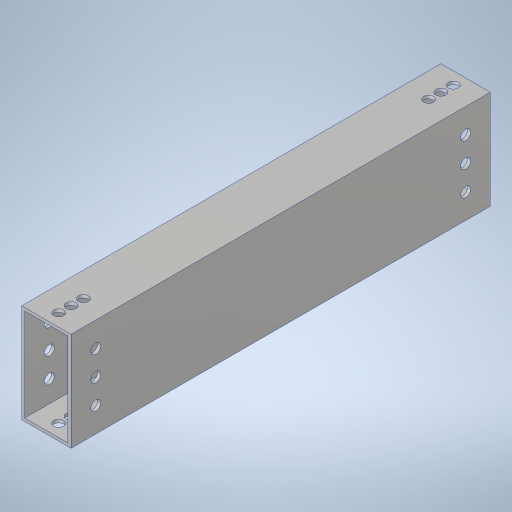
# Autodesk Inventor part: EL2-006
Saved by Autodesk Inventor 2023.4 (Build 274418000, 418)
## iProperties
RuleStatus: InUse
Created: 2025-01-11
Part Number: EL2-006
Material: Aluminum 6061
Document SubType Name: Modeling
Designer: mavericks
Mass: 304.185 g
Surface Area: 718.547 cm^2
Volume: 112.661 cm^3
Density: 2.7 g/cm^3
Appearance: Aluminum - Flat
AfterDocNew0: SHOW
AfterDocOpen0: SHOW
Author: mavericks
Autodesk Inventor part; units mm, degrees
ref_plane "YZ Plane" through (0, 0, 0) normal (1, 0, 0) x (0, 1, 0)
ref_plane "XZ Plane" through (0, 0, 0) normal (0, 1, 0) x (-1, 0, 0)
ref_plane "XY Plane" through (0, 0, 0) normal (0, 0, 1) x (1, 0, 0)
sketch "Sketch1" plane through (0, 0, 0) normal (0, 0, 1) x (1, 0, 0)
  line L0 (-12.7, -25.4) -> (12.7, -25.4)
  line L1 (12.7, -25.4) -> (12.7, 25.4)
  line L2 (12.7, 25.4) -> (-12.7, 25.4)
  line L3 (-12.7, 25.4) -> (-12.7, -25.4)
  line L4 (-12.7, -25.4) -> (12.7, 25.4) construction
  line L5 (12.7, -25.4) -> (-12.7, 25.4) construction
  line L6 (-11.1125, 23.8125) -> (11.1125, 23.8125)
  line L7 (11.1125, 23.8125) -> (11.1125, -23.8125)
  line L8 (11.1125, -23.8125) -> (-11.1125, -23.8125)
  line L9 (-11.1125, -23.8125) -> (-11.1125, 23.8125)
  point P0 (0, 0)
  dimension "width" = 25.4
  dimension "height" = 50.8
  dimension "thickness" = 1.5875
  constraints: 20 end point, 4 parallel, 2 midpoint, 2 perpendicular, 1 horizontal, 3 other
  measures "width" distance of L2.end L1.end
  measures "height" distance of L1.end L0.end
  measures "thickness" distance between parallel lines of L2 L6
extrude "Extrusion1" add sketch "Sketch1" along normal mid plane 215.646
sketch "Sketch2" plane through (12.7, -25.4, 107.823) normal (1, 0, 0) x (0, 0, -1)
  line L0 (0, 49.2125) -> (0, 1.5875) projected
  line L1 (215.646, 50.8) -> (0, 50.8) projected
  line L2 (215.646, 50.8) -> (215.646, 0) construction
  point P0 (107.823, 25.4)
  point P1 (12.7, 38.1)
  point P2 (12.7, 12.7)
  point P3 (12.7, 25.4)
  point P4 (0, 25.4)
  point P5 (202.946, 38.1)
  point P6 (202.946, 12.7)
  point P7 (202.946, 25.4)
  point P8 (215.646, 25.4)
  dimension "d5" = 12.7
  dimension "d6" = 12.7
  dimension "d7" = 12.7
  dimension "d8" = 12.7
  dimension "d9" = 12.7
  dimension "d10" = 12.7
  constraints: 4 vertical alignment, 2 horizontal alignment, 2 midpoint
  measures "d5" distance from line of L1 point (12.7, 38.1)
  measures "d6" distance from line of L0 point (12.7, 25.4)
  measures "d7" distance of point (12.7, 25.4) point (12.7, 12.7)
  measures "d8" distance from line of L2 point (202.946, 38.1)
  measures "d9" distance of point (202.946, 25.4) point (202.946, 38.1)
  measures "d10" distance of point (202.946, 25.4) point (202.946, 12.7)
hole "Hole1" at (12.7, 12.7, 95.123) at (12.7, -12.7, 95.123) at (12.7, 0, 95.123) at (12.7, 12.7, -95.123) at (12.7, 0, -95.123) at (12.7, -12.7, -95.123) direction (-1, 0, 0) diameter 5.1054 end through all clearance for "Flat Head Machine Screw (82)" size "#10" standard "Ansi Unified Screw Threads"
sketch "Sketch3" plane through (-12.7, 25.4, 107.823) normal (0, 1, 0) x (1, 0, 0)
  line L0 (25.4, 0) -> (0, 0) projected
  line L1 (0, 215.646) -> (0, 0) construction
  line L2 (0, 215.646) -> (25.4, 215.646) construction
  point P0 (12.7, 107.823)
  point P1 (12.7, 6.35)
  point P2 (12.7, 12.7)
  point P3 (12.7, 19.05)
  point P4 (12.7, 209.296)
  point P5 (12.7, 202.946)
  point P6 (12.7, 196.596)
  dimension "d18" = 6.35
  dimension "d19" = 6.35
  dimension "d20" = 6.35
  dimension "d21" = 12.7
  dimension "d22" = 6.35
  dimension "d23" = 6.35
  dimension "d24" = 6.35
  constraints: 5 vertical alignment
  measures "d18" distance from line of L0 point (12.7, 6.35)
  measures "d19" distance of point (12.7, 12.7) point (12.7, 6.35)
  measures "d20" distance of point (12.7, 19.05) point (12.7, 12.7)
  measures "d21" distance from line of L1 point (12.7, 6.35)
  measures "d22" distance of point (12.7, 202.946) point (12.7, 196.596)
  measures "d23" distance of point (12.7, 209.296) point (12.7, 202.946)
  measures "d24" distance from line of L2 point (12.7, 209.296)
hole "Hole2" at (0, 25.4, 101.473) at (0, 25.4, 95.123) at (0, 25.4, 88.773) at (0, 25.4, -88.773) at (0, 25.4, -95.123) at (0, 25.4, -101.473) direction (0, -1, 0) diameter 5.1054 end through all clearance for "Flat Head Machine Screw (82)" size "#10" standard "Ansi Unified Screw Threads"
equation "\"d7\" = d5"
equation "\"d8\" = d6"
equation "\"d9\" = d7"
equation "\"d10\" = d7"
equation "\"d20\" = d19"
equation "\"d23\" = d22"
equation "\"d24\" = d23"
body "Solid1"
